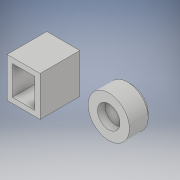
# Autodesk Inventor part: Calculator buttons
Saved by Autodesk Inventor 2018 (Build 220112000, 112)
## iProperties
Created: 2019-09-29
Part Number: Calculator buttons
Material: Generic
Document SubType Name: Modeling
Designer: Hyperspin
Density: 1 g/cm^3
Appearance: Default
Author: Hyperspin
Autodesk Inventor part; units mm, degrees
ref_plane "YZ Plane" through (0, 0, 0) normal (1, 0, 0) x (0, 1, 0)
ref_plane "XZ Plane" through (0, 0, 0) normal (0, 1, 0) x (-1, 0, 0)
ref_plane "XY Plane" through (0, 0, 0) normal (0, 0, 1) x (1, 0, 0)
sketch "Sketch1" plane through (0, 0, 0) normal (0, 0, 1) x (1, 0, 0)
  circle A0 centre (0, 0) radius 2.75
  dimension "d0" = 5.5
  constraints: 1 centre point, 1 coincident
  measures "d0" diameter of A0
extrude "Extrusion1" add sketch "Sketch1" along normal blind 3
sketch "Sketch2" plane through (0, 0, 3) normal (0, 0, 1) x (1, 0, 0)
  circle A0 centre (0, 0) radius 1.5
  dimension "d3" = 3
  constraints: 1 centre point, 1 coincident
  measures "d3" diameter of A0
extrude "Extrusion2" cut sketch "Sketch2" against normal blind 1
chamfer "Chamfer1" distance 0.5 angle 45 1 edges at (-2.75, 0, 0)
sketch "Sketch3" plane through (0, 0, 3) normal (0, 0, 1) x (1, 0, 0)
  line L0 (-9.8546, -0.2887) -> (-12.8546, -0.2887)
  line L1 (-12.8546, -0.2887) -> (-12.8546, -4.1887)
  line L2 (-12.8546, -4.1887) -> (-9.8546, -4.1887)
  line L3 (-9.8546, -4.1887) -> (-9.8546, -0.2887)
  line L4 (-9.1546, -4.8887) -> (-13.5546, -4.8887)
  line L5 (-13.5546, -4.8887) -> (-13.5546, 0.4113)
  line L6 (-13.5546, 0.4113) -> (-9.1546, 0.4113)
  line L7 (-9.1546, 0.4113) -> (-9.1546, -4.8887)
  point P0 (0, 0)
  dimension "d9" = 3
  dimension "d10" = 3.9
  dimension "d11" = 0.7
  constraints: 16 end point, 4 parallel, 2 perpendicular, 1 horizontal, 3 other
  measures "d9" distance of L2.end L1.end
  measures "d10" distance of L0.end L1.end
  measures "d11" distance between parallel lines of L2 L4
extrude "Extrusion3" add sketch "Sketch3" against normal blind 5.8
sketch "Sketch4" plane through (0, 0, -2.8) normal (0, 0, -1) x (-1, 0, 0)
  line L0 (9.8546, -4.1887) -> (9.8546, -0.2887) projected
  line L1 (12.8546, -0.2887) -> (12.8546, -4.1887) projected
  line L2 (12.8546, -4.1887) -> (9.8546, -4.1887) projected
  line L3 (9.8546, -4.1887) -> (9.8546, -0.2887) projected
  line L4 (9.8546, -0.2887) -> (12.8546, -0.2887) projected
  line L5 (9.1546, -4.8887) -> (13.5546, -4.8887) projected
  line L6 (13.5546, -4.8887) -> (13.5546, 0.4113) projected
  line L7 (13.5546, 0.4113) -> (9.1546, 0.4113) projected
  line L8 (9.1546, 0.4113) -> (9.1546, -4.8887) projected
  point P0 (0, 0)
extrude "Extrusion4" add sketch "Sketch4" against normal blind 2 contours L0 L4 L1 L2
chamfer "Chamfer2" distance 0.5 angle 45 4 edges at (-11.3546, -4.8887, -2.8) (-13.5546, -2.2387, -2.8) (-11.3546, 0.4113, -2.8) (-9.1546, -2.2387, -2.8)
body "Solid1"
